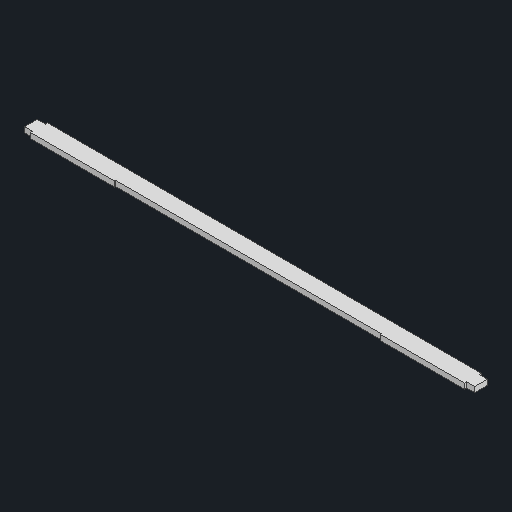
# Autodesk Inventor part: nose
Saved by Autodesk Inventor 2023 (Build 270158030, 158C)
## iProperties
Created: 2022-03-21
Part Number: nose
Material: Generic
Document SubType Name: Modeling
Designer: kardo
Density: 1 g/cm^3
Appearance: Default
Author: kardo
Autodesk Inventor part; units mm, degrees
ref_plane "YZ Plane" through (0, 0, 0) normal (1, 0, 0) x (0, 1, 0)
ref_plane "XZ Plane" through (0, 0, 0) normal (0, 1, 0) x (-1, 0, 0)
ref_plane "XY Plane" through (0, 0, 0) normal (0, 0, 1) x (1, 0, 0)
derived "parameters_frame.ipt"
derived "stencil_frame.ipt"
sketch "sk_joint_locations" plane through (81.12, 0, 0) normal (1, 0, 0) x (0, 1, 0)
  line L0 (0, 0) -> (122.4, 9.6331) construction
  line L1 (36.465, 28.832) -> (112.2, 28.832) construction
  arc A0 (36.465, 28.832) -> (11.22, 28.376) centre (36.465, -670.197) ccw construction
  line L2 (-241.5001, 19.2432) -> (11.22, 28.376) construction
  line L3 (-345, 16.32) -> (-262.2001, 18.586) construction
  arc A1 (-262.2001, 18.586) -> (-241.5001, 19.2432) centre (-326.8578, 2381.2399) ccw construction
  line L4 (-122.4795, 3121.122) -> (270.8781, -1876.9598) construction
  line L5 (-230.0001, 3089.1136) -> (-230.0001, -1866.0023) construction
  line L6 (-114.9999, 3089.1136) -> (-114.9999, -1866.0023) construction
  line L7 (-345, 3089.1136) -> (-345, -1866.0023) construction
  line L8 (0, 3089.1136) -> (0, -1866.0023) construction
  line L9 (529.622, 47.2379) -> (-602.608, 2.7525) construction
  line L10 (-673.1615, -36.5999) -> (647.9226, 67.3717) construction
  line L11 (193.439, 30.0262) -> (193.1249, 38.02) construction
  line L12 (201.1327, 36.2333) -> (201.7624, 28.2333) construction
  line L13 (0, 14.144) -> (121.9006, 15.9783) construction
  line L14 (-230.0001, 45.8224) -> (-230.0001, 19.6588) construction
  line L15 (-345, 37.3935) -> (-345, 16.32) construction
  line L16 (-114.9999, 50.9907) -> (-114.9999, 23.8147) construction
  line L17 (0, 52.89) -> (0, 27.9705) construction
  line L18 (119.1768, 50.5875) -> (119.7216, 43.6656) construction
  line L19 (120.2663, 36.7438) -> (119.7216, 43.6656) construction
  line L20 (120.2663, 36.7438) -> (120.8111, 29.822) construction
  line L21 (120.8111, 29.822) -> (121.3559, 22.9001) construction
  line L22 (121.3559, 22.9001) -> (121.9006, 15.9783) construction
  line L23 (0, 14.144) -> (0, 0) construction
  line L24 (112.2, 37.536) -> (112.2, 28.832) construction
  line L25 (112.2, 35.548) -> (112.2, 30.82) construction
  spline S0 degree 4 poles (-345, 37.3935) (-258.8686, 45.1235) (-172.5923, 49.7074) (-86.3167, 52.89) (0, 52.89) knots 0 0 0 0 0 1 1 1 1 1
  spline S1 degree 3 poles (0, 52.89) (92.8353, 52.89) (195.0311, 49.5089) (255, 36.448) knots 0 0 0 0 1 1 1 1
  spline S2 degree 2 poles (122.4, 9.6331) (190.08, 14.9596) (255, 36.448) knots 0 0 0 1 1 1
  point P0 (-122.4795, 3121.122)
  point P1 (270.8781, -1876.9598)
  point P2 (193.282, 34.0231)
  point P3 (201.4475, 32.2333)
  point P4 (134.9575, 11.3411)
  point P5 (-345, 26.8568)
  point P6 (-230.0001, 32.7406)
  point P7 (-114.9999, 37.4027)
  point P8 (0, 40.4303)
  point P9 (112.2, 33.184)
derived "surface_body.ipt"
sketch "sk_long_inner" plane through (0, 0, 0) normal (1, 0, 0) x (0, 1, 0)
  line L0 (-483, 0) -> (357, 0) construction
  line L1 (-345, 107.6209) -> (-345, -224.5198) construction
  line L2 (-465, 54.4) -> (375, 54.4) construction
  line L3 (0, 107.6209) -> (0, -224.5198) construction
  line L4 (112.2, 107.6209) -> (112.2, -224.5198) construction
  line L5 (11.22, 28.832) -> (112.2, 28.832)
  line L6 (112.2, 37.536) -> (-345, 39.712)
  line L7 (11.22, 28.832) -> (-241.5001, 19.1524)
  line L8 (-241.5001, 19.1524) -> (-345, 16.32)
  line L9 (-345, 16.32) -> (112.2, 16.32) construction
  line L10 (112.2, 16.32) -> (112.2, 28.832) construction
  line L11 (-241.5001, 19.1524) -> (0, 21.3303)
  line L12 (0, 21.3303) -> (112.2, 28.832)
  line L13 (112.2, 37.536) -> (112.2, 28.832)
  line L14 (-114.9999, 107.6209) -> (-114.9999, -224.5198) construction
  line L15 (-230.0001, 107.6209) -> (-230.0001, -224.5198) construction
  line L16 (0, 21.3303) -> (0, 28.4023) construction
  point P0 (0, 0)
  point P1 (112.2, 22.576)
  point P2 (-345, 11.968)
ref_plane "plane_symmetry" through (0, 0, 0) normal (1, 0, 0) x (0, 1, 0)
ref_plane "plane_nose" through (0, 112.2, 0) normal (0, 1, 0) x (-1, 0, 0)
ref_plane "plane_tunnel_right" through (81.12, 0, 0) normal (1, 0, 0) x (0, 1, 0)
ref_plane "plane_cowl_right" through (54.6, 0, 0) normal (1, 0, 0) x (0, 1, 0)
sketch "sk_nose_base" plane through (0, 112.2, 0) normal (0, 1, 0) x (-1, 0, 0)
  line L0 (0, -1280.4843) -> (0, 2991.5273) construction
  line L1 (-81.12, -1280.4843) -> (-81.12, 2991.5273) construction
  line L2 (-81.12, 36.336) -> (-49.6, 36.336)
  line L3 (0, 35.936) -> (0, 30.032)
  line L4 (0, 30.032) -> (-81.12, 30.032)
  line L5 (-81.12, 30.032) -> (-81.12, 30.82)
  line L6 (-81.12, 30.82) -> (-84.12, 30.82)
  line L7 (-84.12, 30.82) -> (-84.12, 35.548)
  line L8 (-84.12, 35.548) -> (-81.12, 35.548)
  line L9 (-81.12, 35.548) -> (-81.12, 36.336)
  line L10 (-54.6, -1280.4843) -> (-54.6, 2991.5273) construction
  line L11 (-49.6, 36.336) -> (-49.6, 35.936)
  line L12 (-49.6, 35.936) -> (0, 35.936)
  point P0 (0, 0)
  point P1 (-81.12, 35.548)
  point P2 (-81.12, 30.82)
  point P3 (0, 37.536)
  point P4 (0, 28.832)
  dimension "d3" = 3
  dimension "d6" = 1.2
  dimension "d7" = 1.2
  dimension "d8" = 1.6
  dimension "d9" = 5
  constraints: 20 end point, 6 collinear, 5 perpendicular, 2 parallel, 2 point on line
  measures "d3" distance between parallel lines of L7 L1
  measures "d6" distance from line of point (0, 37.536) L2
  measures "d7" distance from line of point (0, 28.832) L4
  measures "d8" distance from line of point (0, 37.536) L12
  measures "d9" distance between parallel lines of L10 L11
extrude "thicken" add sketch "sk_nose_base" against normal blind 2
mirror "mirror" about plane through (0, 0, 0) normal (1, 0, 0)
equation "\"d3\" = stringer_thickness"
equation "\"d6\" = shell_thickness"
equation "\"d7\" = shell_thickness"
equation "\"d8\" = cowl_shell_thickness"
equation "\"d9\" = cowl_liner_width"
equation "\"d4\" = bulkhead_thickness"
equation "\"stringer_thickness\" = 3"
equation "\"cowl_liner_width\" = 5"
equation "\"bulkhead_thickness\" = 2"
equation "\"shell_thickness\" = 1.2"
equation "\"cowl_shell_thickness\" = 1.6"
body "Solid1"
